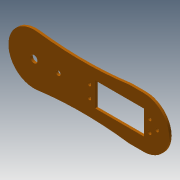
# Autodesk Inventor part: dibond_strana(a)
Saved by Autodesk Inventor 2013 (Build 170138000, 138)
## iProperties
Created: 2013-05-11
Part Number: dibond_strana(a)
Material: Generic
Document SubType Name: Modeling
Designer: idle-rug
Density: 1 g/cm^3
Author: idle-rug
Autodesk Inventor part; units mm, degrees
ref_plane "YZ Plane" through (0, 0, 0) normal (1, 0, 0) x (0, 1, 0)
ref_plane "XZ Plane" through (0, 0, 0) normal (0, 1, 0) x (-1, 0, 0)
ref_plane "XY Plane" through (0, 0, 0) normal (0, 0, 1) x (1, 0, 0)
sketch "Sketch1" plane through (0, 0, 0) normal (0, 1, 0) x (-1, 0, 0)
  circle A0 centre (40, 0) radius 21
  line L0 (-50.5, -21) -> (-38.581, -21)
  line L1 (-50.5, -21) -> (-38.581, -21)
  arc A1 (37.2246, -20.8158) -> (-38.581, -21) centre (0, -300) ccw
  arc A2 (-38.581, 21) -> (37.2246, 20.8158) centre (0, 300) ccw
  line L2 (-50.5, 21) -> (-38.581, 21)
  line L3 (-50.7, -10) -> (-10.5, -10)
  line L4 (-10.5, -10) -> (-10.5, 10)
  line L5 (-10.5, 10) -> (-50.7, 10)
  line L6 (-50.7, 10) -> (-50.7, -10)
  line L7 (-58.1, -10) -> (-3.1, -10)
  line L8 (-3.1, -10) -> (-3.1, 10)
  line L9 (-3.1, 10) -> (-58.1, 10)
  line L10 (-58.1, 10) -> (-58.1, -10)
  line L11 (-10.5, 0) -> (-5.75, 0)
  line L12 (-10.5, -4.95) -> (-10.5, 0)
  line L13 (-10.5, 0) -> (-5.75, 0)
  line L14 (-10.5, 4.95) -> (-10.5, 0)
  circle A3 centre (-5.75, -4.95) radius 1.5
  circle A4 centre (-5.75, 4.95) radius 1.5
  circle A5 centre (-55.45, -4.95) radius 1.5
  circle A6 centre (-55.45, 4.95) radius 1.5
  arc A7 (-50.5, 21) -> (-50.5, -21) centre (-50.5, 0) ccw
  circle A8 centre (40, 0) radius 3
  line L15 (-71.5, 0) -> (-61.5, 0)
  circle A9 centre (-61.5, 0) radius 1.5
  line L16 (40, 0) -> (0, 0)
  circle A10 centre (0, 0) radius 2
  point P0 (-30.6, 0)
  point P1 (-30.6, 0)
  dimension "d2" = 42
  dimension "d11" = 40.2
  dimension "d13" = 55
  dimension "d14" = 20
  dimension "d23" = 3
  dimension "d24" = 6
  dimension "d25" = 40
  dimension "d26" = 10
  dimension "d27" = 3
  dimension "d28" = 40
  dimension "d29" = 4
  constraints: 34 end point, 11 centre point, 9 point on circle, 4 horizontal, 4 parallel, 3 coincident, 2 perpendicular, 2 tangent, 1 collinear
  measures "d2" diameter of A0
  measures "d11" distance of L5.end L4.end
  measures "d13" distance of L9.end L8.end
  measures "d14" distance of L8.end L7.end
  measures "d23" diameter of A6
  measures "d24" diameter of A8
  measures "d25" distance of L16.start L16.end
  measures "d26" distance of L15.start L15.end
  measures "d27" diameter of A9
  measures "d28" distance of L16.start L16.end
  measures "d29" diameter of A10
extrude "Extrusion1" add sketch "Sketch1" along normal blind 2 contours A0 | A0 A1 L0 A7 L2 A2 | L7 L10 L9 L6 | L4 L9 L8 L7
sketch "Sketch2" plane through (0, 0, 0) normal (0, -1, 0) x (1, 0, 0)
  circle A0 centre (0, 0) radius 2 projected
extrude "Extrusion2" add sketch "Sketch2" against normal blind 2
sketch "Sketch3" plane through (0, 0, 0) normal (0, -1, 0) x (1, 0, 0)
  arc A0 (-37.2246, 20.8158) -> (-37.2246, -20.8158) centre (-40, 0) ccw projected
  line L0 (38.581, 21) -> (50.5, 21) projected
  line L1 (-40, 0) -> (-20, 0)
  circle A1 centre (-20, 0) radius 2
  point P0 (0, 0)
  dimension "d34" = 20
  dimension "d35" = 4
  constraints: 2 end point, 1 centre point, 1 coincident, 1 parallel
  measures "d34" distance of L1.start L1.end
  measures "d35" diameter of A1
extrude "Extrusion3" cut sketch "Sketch3" against normal blind 2
body "Solid1"
